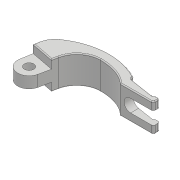
# Autodesk Inventor part: Global Truss 5035-2B P2
Saved by Autodesk Inventor 2018 (Build 220112000, 112)
## iProperties
Created: 2021-01-29
Part Number: Global Truss 5035-2B P2
Material: Generic
Document SubType Name: Modeling
Designer: production
Density: 1 g/cm^3
Appearance: Default
Author: production
Autodesk Inventor part; units mm, degrees
ref_plane "YZ Plane" through (0, 0, 0) normal (1, 0, 0) x (0, 1, 0)
ref_plane "XZ Plane" through (0, 0, 0) normal (0, 1, 0) x (-1, 0, 0)
ref_plane "XY Plane" through (0, 0, 0) normal (0, 0, 1) x (1, 0, 0)
sketch "Sketch1" plane through (0, 0, 0) normal (0, 0, 1) x (1, 0, 0)
  circle A0 centre (0, 0) radius 12
  arc A1 (73.5905, 37) -> (-7.4095, 27.0838) centre (40, -24.3981) ccw
  arc A2 (40, 35.588) -> (15.5254, 15.6865) centre (40, 10.588) ccw
  line L0 (107.5905, 24) -> (107.5905, 31)
  line L1 (107.5905, 31) -> (102.5905, 31)
  line L2 (102.5905, 31) -> (102.5905, 29.5)
  line L3 (102.5905, 29.5) -> (73.5905, 34)
  line L4 (107.5905, 24) -> (72.5905, 24)
  line L5 (73.5905, 34) -> (73.5905, 37)
  line L6 (-11.8177, 2.0838) -> (-7.4095, 27.0838)
  line L7 (12, 0) -> (12.2576, 0)
  line L8 (11.7478, -2.4473) -> (15.5254, 15.6865)
  ellipse E0 centre (40, 10.588) end of major axis (78.6183, 10.588) minor radius 25 (72.5905, 24) -> (40, 35.588) ccw
  dimension "d0" = 24
  dimension "d2" = 50
  dimension "d5" = 10
  dimension "d6" = 5.5
  dimension "d8" = 7
  dimension "d9" = 5
  dimension "d11" = 3
  dimension "d12" = 24
  dimension "d13" = 115
  dimension "d14" = 100
  dimension "d15" = 25
  dimension "d16" = 34
  dimension "d18" = 40
  dimension "d19" = 10
  dimension "d26" = 35
  constraints: 18 end point, 7 point on circle, 3 centre point, 3 horizontal, 3 tangent, 2 coincident, 2 vertical, 1 perpendicular, 1 point on line, 1 vertical alignment, 5 other
  measures "d0" diameter of A0
  measures "d2" diameter of A2
  measures "d5" distance from line of L4 L3.end
  measures "d6" distance from line of L4 L2.end
  measures "d8" distance between parallel lines of L4 L1
  measures "d9" distance of L0.end L1.end
  measures "d11" distance of L3.end L5.end
  measures "d12" distance from line of L4 A0.centre
  measures "d13" distance from line of L6.end L0
  measures "d14" angle of L4 L6
  measures "d15" vertical distance of L6.start L6.end
  measures "d16" distance between parallel lines of L5 L0
  measures "d18" horizontal distance of A2.centre A0.centre
  measures "d26" distance of L4.end L0.start
extrude "Extrusion2" add sketch "Sketch1" along normal mid plane 30
fillet "Fillet1" radius 2 6 edges at (107.5905, 31, 0) (107.5905, 24, 0) (73.5905, 34, 0) (73.5905, 37, 0) (102.5905, 29.5, 0) (102.5905, 31, 0)
fillet "Fillet2" radius 20 1 edges at (-7.4095, 27.0838, 0)
sketch "Sketch2" plane through (72.5905, 24, -15) normal (0, -1, 0) x (1, 0, 0)
  line L0 (11, 15) -> (35, 15) construction
  line L1 (11, 8.25) -> (35, 8.25)
  line L2 (35, 21.75) -> (11, 21.75)
  arc A0 (11, 21.75) -> (11, 8.25) centre (11, 15) ccw
  arc A1 (35, 8.25) -> (35, 21.75) centre (35, 15) ccw
  line L3 (33, 30) -> (33, 0) projected
  line L4 (35, 0) -> (35, 30) projected
  point P0 (-72.5905, 15)
  point P1 (23, 15)
  point P2 (33, 15)
  dimension "d27" = 13.5
  dimension "d28" = 24
  constraints: 8 end point, 4 point on circle, 4 tangent, 3 midpoint, 2 centre point, 1 horizontal, 1 horizontal alignment, 1 parallel
  measures "d27" distance between parallel lines of L1 L2
  measures "d28" distance from line of L4 L0.start
extrude "Extrusion3" cut sketch "Sketch2" against normal through all
sketch "Sketch3" plane through (0, 0, 15) normal (0, 0, 1) x (1, 0, 0)
  line L0 (-9.7015, 14.0852) -> (14.2331, 9.4831)
  line L1 (11.7478, -2.4473) -> (15.5254, 15.6865) projected
  line L2 (-8.6958, 19.7888) -> (-11.8177, 2.0838) projected
  arc A0 (11.7478, -2.4473) -> (-11.8177, 2.0838) centre (0, 0) ccw projected
  line L3 (2.2658, 11.7841) -> (0, 0)
  arc A1 (-11.8177, 2.0838) -> (11.7478, -2.4473) centre (0, 0) ccw projected
  line L4 (-11.8177, 2.0838) -> (-8.6958, 19.7888) projected
  line L5 (-9.7015, 14.0852) -> (-11.8177, 2.0838)
  line L6 (14.2331, 9.4831) -> (11.7478, -2.4473)
  dimension "d31" = 90
  dimension "d32" = 12
  constraints: 8 end point, 2 point on line, 2 tangent, 1 collinear, 1 midpoint
  measures "d31" angle of L3 L0
  measures "d32" distance from line of L3.end L0
extrude "Extrusion4" cut sketch "Sketch3" against normal blind 9
mirror "Mirror1" about plane through (0, 0, 0) normal (0, 0, 1) of "Extrusion4"
sketch "Sketch4" plane through (0, 0, -6) normal (0, 0, -1) x (-0.9820122, 0.1888173, 0)
  circle A0 centre (0, 0) radius 5
  dimension "d35" = 10
  constraints: 1 centre point, 1 coincident
  measures "d35" diameter of A0
extrude "Extrusion5" cut sketch "Sketch4" against normal through all
fillet "Fillet3" radius 1 30 edges at (-5.9106, 26.9938, 15) (-9.1987, 16.937, 15) (73.302, 36.8375, 15) (73.5905, 35.7582, 15) (87.869, 31.7844, 15) (107.0047, 24.5858, 15) (107.0047, 30.4142, 15) (104.6001, 31, 15) (107.5905, 27.5, 15) (89.0905, 24, 15) (35.2562, 45.427, 15) (24.2276, 29.9846, 15) (14.8793, 12.5848, 15) (58.5914, 32.5003, 15) (2.2658, 11.7841, 15) (-9.1987, 16.937, -15) (35.2562, 45.427, -15) (73.302, 36.8375, -15) (73.5905, 35.7582, -15) (87.869, 31.7844, -15) (107.0047, 24.5858, -15) (107.0047, 30.4142, -15) (104.6001, 31, -15) (107.5905, 27.5, -15) (89.0905, 24, -15) (-5.9106, 26.9938, -15) (2.2658, 11.7841, -15) (14.8793, 12.5848, -15) (58.5914, 32.5003, -15) (24.2276, 29.9846, -15)
body "Solid2"
